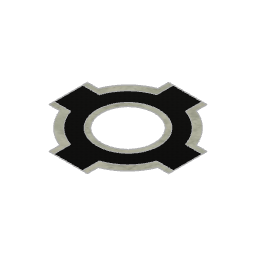
_Room Dimensions v1_Roundabout 52 id.9af43ff4-770a-4ec2-8674-011271ecb3cc (Autodesk Fusion 360 design; units mm, degrees)
Autodesk Fusion 360 part; units mm, degrees
note: some values were not read from the file. Set by a fixed rule: which sketch regions a step uses.
sketch "Sketch1" plane through (0, 0, 0) normal (0, 0, 1) x (1, 0, 0)
  circle A0 centre (-5079.9999, 2540) radius 660.4
  circle A1 centre (-5079.9999, 2540) radius 965.2
  line L0 (-6349.9999, 2844.8) -> (-3809.9999, 2844.8)
  line L1 (-3809.9999, 2844.8) -> (-3809.9999, 2235.2)
  line L2 (-3809.9999, 2235.2) -> (-6349.9999, 2235.2)
  line L3 (-6349.9999, 2235.2) -> (-6349.9999, 2844.8)
  line L4 (-6349.9999, 2844.8) -> (-3809.9999, 2235.2) construction
  line L5 (-3809.9999, 2844.8) -> (-6349.9999, 2235.2) construction
  line L6 (-4775.1999, 3810) -> (-5384.7999, 3810)
  line L7 (-5384.7999, 3810) -> (-5384.7999, 1270)
  line L8 (-5384.7999, 1270) -> (-4775.1999, 1270)
  line L9 (-4775.1999, 1270) -> (-4775.1999, 3810)
  line L10 (-4775.1999, 3810) -> (-5384.7999, 1270) construction
  line L11 (-5384.7999, 3810) -> (-4775.1999, 1270) construction
  line L12 (-6349.9999, 2235.2) -> (-3845.6793, 2235.2)
  line L13 (-3845.6793, 2235.2) -> (-3845.6793, 2133.6)
  line L14 (-3845.6793, 2133.6) -> (-6349.9999, 2133.6)
  line L15 (-6349.9999, 2133.6) -> (-6349.9999, 2235.2)
  line L16 (-6349.9999, 2844.8) -> (-3809.9999, 2844.8)
  line L17 (-3809.9999, 2844.8) -> (-3809.9999, 2946.4)
  line L18 (-3809.9999, 2946.4) -> (-6349.9999, 2946.4)
  line L19 (-6349.9999, 2946.4) -> (-6349.9999, 2844.8)
  line L20 (-5384.7999, 3810) -> (-5486.3999, 3810)
  line L21 (-5486.3999, 3810) -> (-5486.3999, 1270)
  line L22 (-5486.3999, 1270) -> (-5384.7999, 1270)
  line L23 (-5384.7999, 1270) -> (-5384.7999, 3810)
  line L24 (-4775.1999, 1270) -> (-4673.5999, 1270)
  line L25 (-4673.5999, 1270) -> (-4673.5999, 3809.9999)
  line L26 (-4673.5999, 3809.9999) -> (-4775.1999, 3809.9999)
  line L27 (-4775.1999, 3809.9999) -> (-4775.1999, 1270)
  circle A2 centre (-5079.9999, 2540) radius 558.8
  circle A3 centre (-5079.9999, 2540) radius 1117.6
  line L28 (-3845.6793, 2133.6) -> (-3809.9999, 2133.6)
  line L29 (-3809.9999, 2133.6) -> (-3809.9999, 2235.2)
  line L30 (-3809.9999, 2235.2) -> (-3845.6793, 2235.2)
  line L31 (-3845.6793, 2235.2) -> (-3845.6793, 2133.6)
  point P0 (-5079.9999, 2540)
  point P1 (-5079.9999, 2540)
  dimension "d1" = 1320.8
  dimension "d2" = 1930.4
  dimension "d3" = 2540
  dimension "d4" = 609.6
  dimension "d5" = 609.6
  dimension "d6" = 2540
  dimension "d7" = 101.6
  dimension "d8" = 101.6
  dimension "d9" = 101.6
  dimension "d10" = 101.6
  dimension "d11" = 1117.6
  dimension "d12" = 2235.2
  constraint concentric A0 A1
  constraint horizontal L0
  constraint perpendicular L0 L1
  constraint parallel L0 L2
  constraint parallel L1 L3
  constraint coincident L4 P1
  constraint coincident L5 P1
  constraint coincident P0 A0.centre
  constraint horizontal L6
  constraint perpendicular L6 L7
  constraint parallel L6 L8
  constraint parallel L7 L9
  constraint coincident L10 P1
  constraint coincident L11 P1
  constraint coincident P1 P0
  constraint horizontal L12
  constraint vertical L13
  constraint horizontal L14
  constraint vertical L15
  constraint horizontal L16
  constraint vertical L17
  constraint horizontal L18
  constraint vertical L19
  constraint horizontal L20
  constraint vertical L21
  constraint horizontal L22
  constraint vertical L23
  constraint horizontal L24
  constraint vertical L25
  constraint horizontal L26
  constraint vertical L27
  constraint concentric A0 A2
  constraint concentric A1 A3
  constraint horizontal L28
  constraint vertical L29
  constraint horizontal L30
  constraint vertical L31
  measures "d1" diameter of A0
  measures "d2" diameter of A1
  measures "d3" distance of L1.end L2.end
  measures "d4" distance of L0.end L1.end
  measures "d5" distance of L7.end L8.end
  measures "d6" distance of L6.end L7.end
  measures "d7" distance of L2.end L14.end
  measures "d8" distance of L0.start L18.end
  measures "d9" distance of L6.end L20.end
  measures "d10" distance of L8.end L24.end
  measures "d11" diameter of A2
  measures "d12" diameter of A3
extrude "Extrude1" add sketch "Sketch1" along normal blind 6.35 contours A0 A1 L0 L2 L12 L16 | A0 A1 L0 L16 L18 | A0 A1 L2 L12 L14 | A0 A1 L18 L25 | A1 L0 L2 L12 L16 A3 | A0 A1 L14 L25 | A0 A1 L9 L25 L27 | L0 L1 L2 L12 L16 A3 L30 | A0 A1 L9 L25 L27 | A0 A1 L7 L9 L23 L27 | A0 A1 L7 L9 L23 L27 | A0 A1 L7 L21 L23 | A1 L7 L9 L23 L27 A3 | A0 A1 L7 L21 L23 | A1 L7 L9 L23 L27 A3 | A0 A1 L18 L21 | L6 L7 L9 L23 L27 A3 | A0 A1 L14 L21 | L7 L8 L9 L23 L27 A3 | A0 A1 L0 L16 L18 | A0 A1 L2 L12 L14 | A0 A1 L0 L2 L12 L16 | A1 L0 L2 L12 L16 A3 | L0 L2 L3 L12 L16 A3
extrude "Extrude2" add sketch "Sketch1" along normal blind 6.096 contours A0 L0 L2 L12 L16 A2 | A0 L0 L16 L18 L25 A2 | A0 L2 L12 L14 L25 A2 | A0 L18 L25 | A1 L0 L16 L18 A3 | A0 L14 L25 | A1 L2 L12 L14 A3 | A0 L9 L18 L25 L27 A2 | A1 L18 L25 A3 | L0 L16 L17 L18 A3 | A0 L9 L14 L25 L27 A2 | A1 L14 L25 A3 | L2 L12 L13 L14 A3 L31 | A0 L7 L9 L23 L27 A2 | A1 L9 L25 L27 A3 | A0 L7 L9 L23 L27 A2 | A1 L9 L25 L27 A3 | A0 L7 L18 L21 L23 A2 | L9 L25 L26 L27 A3 | A0 L7 L14 L21 L23 A2 | L9 L24 L25 L27 A3 | A0 L18 L21 | A1 L7 L21 L23 A3 | A0 L14 L21 | A1 L7 L21 L23 A3 | A0 L0 L16 L18 L21 A2 | A1 L18 L21 A3 | L7 L20 L21 L23 A3 | A0 L0 L2 L12 L16 A2 | A0 L2 L12 L14 L21 A2 | A1 L14 L21 A3 | L7 L21 L22 L23 A3 | A1 L0 L16 L18 A3 | A1 L2 L12 L14 A3 | L0 L16 L18 L19 A3 | L2 L12 L14 L15 A3
extrude "Extrude3" add sketch "Sketch1" along normal blind 6.096 contours L2 L13 L28 L29 L30 L31
